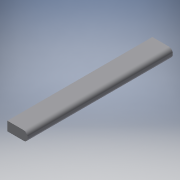
# Autodesk Inventor part: GuideArm
Saved by Autodesk Inventor 2018 (Build 220112000, 112)
## iProperties
Created: 2017-12-14
Part Number: GuideArm
Material: Generic
Document SubType Name: Modeling
Designer: reide
Density: 1 g/cm^3
Appearance: Default
Author: reide
Autodesk Inventor part; units mm, degrees
ref_plane "YZ Plane" through (0, 0, 0) normal (1, 0, 0) x (0, 1, 0)
ref_plane "XZ Plane" through (0, 0, 0) normal (0, 1, 0) x (-1, 0, 0)
ref_plane "XY Plane" through (0, 0, 0) normal (0, 0, 1) x (1, 0, 0)
sketch "Sketch1" plane through (0, 0, 0) normal (0, 1, 0) x (-1, 0, 0)
  line L0 (0, 0) -> (0, -4.826)
  line L1 (0, -4.826) -> (9.652, -4.826)
  line L2 (9.652, -4.826) -> (9.652, 0)
  line L3 (9.652, 0) -> (0, 0)
  dimension "d0" = 4.826
  dimension "d1" = 9.652
  constraints: 8 end point, 2 vertical, 1 horizontal, 1 perpendicular
  measures "d0" distance of L0.start L0.end
  measures "d1" distance of L0.end L1.end
extrude "Extrusion1" add sketch "Sketch1" along normal blind 76.2
fillet "Fillet1" radius 2 2 edges at (0, 38.1, 0) (0, 38.1, -4.826)
sketch "Sketch2" plane through (-9.652, 0, -4.826) normal (-1, 0, 0) x (0, 0, 1)
  line L0 (4.826, 0) -> (4.826, 76.2) projected
  line L1 (0, 0) -> (0, 76.2) projected
  line L2 (0, 0) -> (4.826, 0) projected
  line L3 (0, 76.2) -> (4.826, 76.2) projected
extrude "Extrusion2" add sketch "Sketch2" along normal blind 1
fillet "Fillet2" radius 1 2 edges at (-10.652, 38.1, -4.826) (-10.652, 38.1, 0)
body "Solid1"
